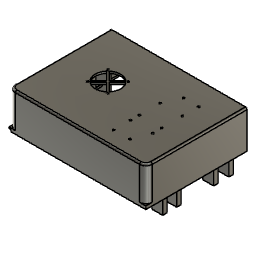
후방 상단 덮개 (Autodesk Fusion 360 design; units mm, degrees)
Autodesk Fusion 360 part; units mm, degrees
note: some values were not read from the file. Set by a fixed rule: which sketch regions a step uses.
sketch "스케치1" plane through (0, 0, 0) normal (0, 0, 1) x (1, 0, 0)
  line L0 (107.5, 79.5) -> (-107.5, 79.5)
  line L1 (-107.5, 79.5) -> (-107.5, -79.5)
  line L2 (-107.5, -79.5) -> (107.5, -79.5)
  line L3 (107.5, -79.5) -> (107.5, 79.5)
  line L4 (107.5, 79.5) -> (-107.5, -79.5) construction
  line L5 (-107.5, 79.5) -> (107.5, -79.5) construction
  line L6 (-107.5, 79.5) -> (-87.5, 79.5)
  line L7 (-87.5, 79.5) -> (-87.5, -79.5)
  line L8 (-87.5, -79.5) -> (-107.5, -79.5)
  line L9 (-107.5, -79.5) -> (-107.5, 79.5)
  line L10 (107.5, 79.5) -> (87.5, 79.5)
  line L11 (87.5, 79.5) -> (87.5, -79.5)
  line L12 (87.5, -79.5) -> (107.5, -79.5)
  line L13 (107.5, -79.5) -> (107.5, 79.5)
  line L14 (-107.5, 79.5) -> (-107.5, 69.5)
  line L15 (0, 0) -> (0, 10)
  line L16 (-107.5, 69.5) -> (-87.5, 69.5)
  line L17 (-87.5, 69.5) -> (-87.5, 21.5)
  line L18 (-87.5, 21.5) -> (-107.5, 21.5)
  line L19 (-107.5, 21.5) -> (-107.5, 69.5)
  line L20 (-97.5, 45.5) -> (-97.5, 57.5)
  line L21 (-107.5, 61) -> (-87.5, 61)
  line L22 (-87.5, 61) -> (-87.5, 54)
  line L23 (-87.5, 54) -> (-107.5, 54)
  line L24 (-107.5, 54) -> (-107.5, 61)
  line L25 (-107.5, 61) -> (-87.5, 54) construction
  line L26 (-87.5, 61) -> (-107.5, 54) construction
  line L27 (-97.5, 45.5) -> (-97.5, 33.5)
  line L28 (-87.5, 37) -> (-107.5, 37)
  line L29 (-107.5, 37) -> (-107.5, 30)
  line L30 (-107.5, 30) -> (-87.5, 30)
  line L31 (-87.5, 30) -> (-87.5, 37)
  line L32 (-87.5, 37) -> (-107.5, 30) construction
  line L33 (-107.5, 37) -> (-87.5, 30) construction
  circle A0 centre (-97.5, 57.5) radius 1.6
  circle A1 centre (-97.5, 33.5) radius 1.6
  line L34 (-107.5, -79.5) -> (-107.5, -59.5)
  line L35 (-107.5, -59.5) -> (-87.5, -59.5)
  line L36 (-87.5, -59.5) -> (-87.5, -11.5)
  line L37 (-87.5, -11.5) -> (-107.5, -11.5)
  line L38 (-107.5, -11.5) -> (-107.5, -59.5)
  line L39 (-97.5, -35.5) -> (-97.5, -24.5)
  line L40 (-97.5, -35.5) -> (-97.5, -46.5)
  line L41 (-107.5, -21) -> (-87.5, -21)
  line L42 (-87.5, -21) -> (-87.5, -28)
  line L43 (-87.5, -28) -> (-107.5, -28)
  line L44 (-107.5, -28) -> (-107.5, -21)
  line L45 (-107.5, -21) -> (-87.5, -28) construction
  line L46 (-87.5, -21) -> (-107.5, -28) construction
  line L47 (-87.5, -43) -> (-107.5, -43)
  line L48 (-107.5, -43) -> (-107.5, -50)
  line L49 (-107.5, -50) -> (-87.5, -50)
  line L50 (-87.5, -50) -> (-87.5, -43)
  line L51 (-87.5, -43) -> (-107.5, -50) construction
  line L52 (-107.5, -43) -> (-87.5, -50) construction
  circle A2 centre (-97.5, -24.5) radius 1.6
  circle A3 centre (-97.5, -46.5) radius 1.6
  line L53 (107.5, 79.5) -> (104.5, 79.5)
  line L54 (104.5, 79.5) -> (104.5, 76.5)
  line L55 (104.5, 76.5) -> (107.5, 76.5)
  line L56 (107.5, 76.5) -> (107.5, 79.5)
  line L57 (-107.5, -79.5) -> (-104.5, -79.5)
  line L58 (-104.5, -79.5) -> (-104.5, -76.5)
  line L59 (-104.5, -76.5) -> (-107.5, -76.5)
  line L60 (-107.5, -76.5) -> (-107.5, -79.5)
  line L61 (-104.5, -76.5) -> (104.5, -76.5)
  line L62 (104.5, -76.5) -> (104.5, 76.5)
  line L63 (104.5, 76.5) -> (-104.5, 76.5)
  line L64 (-104.5, 76.5) -> (-104.5, -76.5)
  line L65 (107.5, 61) -> (87.5, 61)
  line L66 (87.5, 61) -> (87.5, 54)
  line L67 (87.5, 54) -> (107.5, 54)
  line L68 (107.5, 54) -> (107.5, 61)
  circle A4 centre (97.5, 57.5) radius 1.6
  line L69 (107.5, 30) -> (87.5, 30)
  line L70 (87.5, 30) -> (87.5, 37)
  line L71 (107.5, 37) -> (107.5, 30)
  line L72 (87.5, 37) -> (107.5, 37)
  circle A5 centre (97.5, 33.5) radius 1.6
  line L73 (107.5, -50) -> (87.5, -50)
  line L74 (87.5, -50) -> (87.5, -43)
  line L75 (107.5, -43) -> (107.5, -50)
  line L76 (87.5, -43) -> (107.5, -43)
  circle A6 centre (97.5, -46.5) radius 1.6
  line L77 (107.5, -21) -> (87.5, -21)
  line L78 (87.5, -21) -> (87.5, -28)
  line L79 (107.5, -28) -> (107.5, -21)
  line L80 (87.5, -28) -> (107.5, -28)
  circle A7 centre (97.5, -24.5) radius 1.6
  line L81 (-104.5, 76.5) -> (-104.5, 79.5)
  point P0 (-97.5, 57.5)
  point P1 (-97.5, 33.5)
  point P2 (-97.5, -24.5)
  point P3 (-97.5, -46.5)
  dimension "d1" = 215
  dimension "d2" = 159
  dimension "d3" = 20
  dimension "d4" = 20
  dimension "d5" = 10
  dimension "d6" = 48
  dimension "d7" = 12
  dimension "d8" = 7
  dimension "d9" = 12
  dimension "d10" = 7
  dimension "d11" = 3.2
  dimension "d12" = 3.2
  dimension "d13" = 20
  dimension "d14" = 48
  dimension "d15" = 11
  dimension "d16" = 11
  dimension "d17" = 7
  dimension "d18" = 7
  dimension "d19" = 3.2
  dimension "d20" = 3.2
  dimension "d21" = 3
  dimension "d22" = 3
  dimension "d23" = 3
  dimension "d24" = 3
  constraint horizontal L0
  constraint perpendicular L0 L1
  constraint parallel L0 L2
  constraint parallel L1 L3
  constraint coincident L4 L15.start
  constraint coincident L5 L15.start
  constraint coincident L15.start origin
  constraint horizontal L6
  constraint vertical L7
  constraint horizontal L8
  constraint vertical L9
  constraint coincident L2 L7.end
  constraint horizontal L10
  constraint vertical L11
  constraint horizontal L12
  constraint vertical L13
  constraint perpendicular L6 L14
  constraint parallel L7 L15
  constraint horizontal L16
  constraint vertical L17
  constraint horizontal L18
  constraint vertical L19
  constraint perpendicular L18 L20
  constraint horizontal L21
  constraint perpendicular L21 L22
  constraint parallel L21 L23
  constraint parallel L22 L24
  constraint coincident L25 P0
  constraint coincident L26 P0
  constraint coincident P0 L20.end
  constraint parallel L20 L27
  constraint horizontal L28
  constraint perpendicular L28 L29
  constraint parallel L28 L30
  constraint parallel L29 L31
  constraint coincident L32 P1
  constraint coincident L33 P1
  constraint coincident P1 L27.end
  constraint perpendicular L2 L34
  constraint horizontal L35
  constraint vertical L36
  constraint horizontal L37
  constraint vertical L38
  constraint perpendicular L35 L39
  constraint perpendicular L37 L40
  constraint horizontal L41
  constraint perpendicular L41 L42
  constraint parallel L41 L43
  constraint parallel L42 L44
  constraint coincident L45 P2
  constraint coincident L46 P2
  constraint coincident P2 L39.end
  constraint horizontal L47
  constraint perpendicular L47 L48
  constraint parallel L47 L49
  constraint parallel L48 L50
  constraint coincident L51 P3
  constraint coincident L52 P3
  constraint coincident P3 L40.end
  constraint horizontal L53
  constraint vertical L54
  constraint horizontal L55
  constraint vertical L56
  constraint horizontal L57
  constraint vertical L58
  constraint horizontal L59
  constraint vertical L60
  constraint horizontal L61
  constraint vertical L62
  constraint horizontal L63
  constraint vertical L64
  constraint symmetric L15 L21.start L65.start
  constraint symmetric L15 L21.end L65.end
  constraint symmetric L15 L22.end L66.end
  constraint symmetric L15 L23.end L67.end
  constraint symmetric L15 L28.start L70.end
  constraint symmetric L15 L28.end L71.start
  constraint symmetric L15 L29.end L69.start
  constraint symmetric L15 L30.end L69.end
  constraint symmetric L15 A0 A4
  constraint symmetric L15 A1 A5
  constraint symmetric L15 L41.start L77.start
  constraint symmetric L15 L41.end L77.end
  constraint symmetric L15 L42.end L78.end
  constraint symmetric L15 L43.end L79.start
  constraint symmetric L15 L47.start L74.end
  constraint symmetric L15 L47.end L75.start
  constraint symmetric L15 L48.end L73.start
  constraint symmetric L15 L49.end L73.end
  constraint symmetric L15 A2 A7
  constraint symmetric L15 A3 A6
  constraint coincident L6 L81.end
  measures "d1" distance of L1.end L2.end
  measures "d2" distance of L0.end L1.end
  measures "d3" distance of L0.end L6.end
  measures "d4" distance of L0.start L10.end
  measures "d5" distance of L0.end L14.end
  measures "d6" distance of L14.end L18.end
  measures "d7" distance of L20.start P0
  measures "d8" distance of L21.end L22.end
  measures "d9" distance of L20.start P1
  measures "d10" distance of L28.end L29.end
  measures "d11" diameter of A0
  measures "d12" diameter of A1
  measures "d13" distance of L1.end L34.end
  measures "d14" distance of L34.end L37.end
  measures "d15" distance of L39.start P2
  measures "d16" distance of L39.start P3
  measures "d17" distance of L41.end L42.end
  measures "d18" distance of L47.end L48.end
  measures "d19" diameter of A2
  measures "d20" diameter of A3
  measures "d21" distance of L0.start L53.end
  measures "d22" distance of L0.start L55.end
  measures "d23" distance of L1.end L57.end
  measures "d24" distance of L1.end L59.end
extrude "돌출1" add sketch "스케치1" along normal blind 59 contours L0 L3 L10 L13 L53 L54 L55 L56 | L3 L13 L55 L62 L65 | L3 L13 L62 L65 L67 L68 | L3 L13 L62 L67 L72 | L0 L1 L6 L9 L14 L16 L64 L81 | L3 L13 L62 L69 L71 L72 | L3 L13 L62 L69 L77 | L1 L9 L16 L19 L21 L64 | L3 L13 L62 L77 L79 L80 | L1 L9 L19 L21 L23 L24 L64 | L3 L13 L62 L76 L80 | L1 L9 L19 L23 L28 L64 | L3 L13 L62 L73 L75 L76 | L1 L9 L19 L28 L29 L30 L64 | L2 L3 L11 L12 L13 L61 L62 L73 | L1 L9 L18 L19 L30 L64 | L1 L9 L18 L37 L64 | L2 L7 L11 L61 | L1 L9 L37 L38 L41 L64 | L2 L7 L8 L58 L61 | L1 L9 L38 L41 L43 L44 L64 | L1 L2 L8 L9 L34 L57 L58 L59 L60 | L1 L9 L38 L43 L47 L64 | L1 L9 L34 L35 L59 L64 | L1 L9 L38 L47 L48 L49 L64 | L1 L9 L35 L38 L49 L64
sketch "스케치2" plane through (0, 0, 0) normal (0, 0, -1) x (1, 0, 0)
  line L0 (-104.5, -76.5) -> (-104.5, 76.5)
  line L1 (-104.5, 76.5) -> (104.5, 76.5)
  line L2 (104.5, 76.5) -> (104.5, -79.5)
  line L3 (104.5, -79.5) -> (107.5, -79.5)
  line L4 (107.5, -79.5) -> (107.5, 79.5)
  line L5 (107.5, 79.5) -> (-107.5, 79.5)
  line L6 (-107.5, 79.5) -> (-107.5, -79.5)
  line L7 (-107.5, -79.5) -> (-104.5, -79.5)
  line L8 (-104.5, -79.5) -> (-104.5, -76.5)
  line L9 (-104.5, 76.5) -> (-94.5, 76.5)
  line L10 (-94.5, 76.5) -> (-94.5, -79.5)
  line L11 (-94.5, -79.5) -> (-104.5, -79.5)
  line L12 (-104.5, -79.5) -> (-104.5, 76.5)
  line L13 (104.5, 76.5) -> (94.5, 76.5)
  line L14 (94.5, 76.5) -> (94.5, -79.5)
  line L15 (94.5, -79.5) -> (104.5, -79.5)
  line L16 (104.5, -79.5) -> (104.5, 76.5)
  dimension "d27" = 10
  dimension "d28" = 10
  constraint horizontal L9
  constraint vertical L10
  constraint horizontal L11
  constraint vertical L12
  constraint coincident L0.end L1.start
  constraint horizontal L13
  constraint vertical L14
  constraint horizontal L15
  constraint vertical L16
  constraint coincident L1.end L2.start
  measures "d27" distance of L0.end L9.end
  measures "d28" distance of L1.end L13.end
extrude "돌출2" add sketch "스케치2" against normal blind 3 contours L0 L1 L8 L9 L10 L11 L12 | L1 L2 L13 L14 L15 L16
extrude "돌출3" add sketch "스케치1" against normal blind 24 contours L11 L62 L65 L66 L67 | L11 L62 L69 L70 L72 | L7 L17 L21 L22 L23 L64 | L11 L62 L77 L78 L80 | L7 L17 L28 L30 L31 L64 | L11 L62 L73 L74 L76 | L7 L36 L41 L42 L43 L64 | L7 L36 L47 L49 L50 L64
extrude "돌출4" add sketch "스케치1" against normal blind 21.8 contours A0 | A1 | A2 | A3 | A4 | A5 | A6 | A7
sketch "스케치3" plane through (104.5, 0, 0) normal (-1, 0, 0) x (0, -1, 0)
  line L0 (-79.5, 3) -> (76.5, 3)
  line L1 (76.5, 3) -> (76.5, 59)
  line L2 (76.5, 59) -> (-79.5, 59)
  line L3 (-79.5, 59) -> (-79.5, 3)
  line L4 (76.5, 59) -> (-79.5, 59)
  line L5 (-79.5, 59) -> (-79.5, 56)
  line L6 (-79.5, 56) -> (76.5, 56)
  line L7 (76.5, 56) -> (76.5, 59)
  dimension "d35" = 3
  constraint horizontal L4
  constraint vertical L5
  constraint horizontal L6
  constraint vertical L7
  constraint coincident L1.end L2.start
  measures "d35" distance of L1.end L6.end
extrude "돌출5" add sketch "스케치3" along normal blind 212 contours L1 L2 L3 L4 L5 L6 L7
extrude "돌출6" add 8 faces at (89.8333, 58.6667, 0) (89.8333, 34.6667, 0) (92.1667, -23.3333, 0) (92.1667, -47.6667, 0) (-89.8333, 58.6667, 0) (-89.8333, 32.3333, 0) (-92.1667, -45.3333, 0) (-92.1667, -25.6667, 0) along direction (0, 0, 1) blind 3
sketch "스케치6" plane through (0, 0, 3) normal (0, 0, 1) x (-1, 0, 0)
  line L0 (94.5, -79.5) -> (104.5, -79.5)
  line L1 (104.5, -79.5) -> (104.5, -76.5)
  line L2 (104.5, -76.5) -> (104.5, 76.5)
  line L3 (104.5, 76.5) -> (94.5, 76.5)
  line L4 (94.5, 76.5) -> (94.5, 50)
  line L5 (94.5, 50) -> (87.5, 50)
  line L6 (87.5, 50) -> (87.5, 43)
  line L7 (87.5, 43) -> (94.5, 43)
  line L8 (94.5, 43) -> (94.5, 28)
  line L9 (94.5, 28) -> (87.5, 28)
  line L10 (87.5, 28) -> (87.5, 21)
  line L11 (87.5, 21) -> (94.5, 21)
  line L12 (94.5, 21) -> (94.5, -30)
  line L13 (94.5, -30) -> (87.5, -30)
  line L14 (87.5, -30) -> (87.5, -37)
  line L15 (87.5, -37) -> (94.5, -37)
  line L16 (94.5, -37) -> (94.5, -54)
  line L17 (94.5, -54) -> (87.5, -54)
  line L18 (87.5, -54) -> (87.5, -61)
  line L19 (87.5, -61) -> (94.5, -61)
  line L20 (94.5, -61) -> (94.5, -79.5)
  line L21 (87.5, 50) -> (104.5, 50)
  line L22 (104.5, 50) -> (104.5, 43)
  line L23 (104.5, 43) -> (87.5, 43)
  line L24 (87.5, 43) -> (87.5, 50)
  line L25 (87.5, 28) -> (104.5, 28)
  line L26 (104.5, 28) -> (104.5, 21)
  line L27 (104.5, 21) -> (87.5, 21)
  line L28 (87.5, 21) -> (87.5, 28)
  line L29 (87.5, -30) -> (104.5, -30)
  line L30 (104.5, -30) -> (104.5, -37)
  line L31 (104.5, -37) -> (87.5, -37)
  line L32 (87.5, -37) -> (87.5, -30)
  line L33 (87.5, -54) -> (104.5, -54)
  line L34 (104.5, -54) -> (104.5, -61)
  line L35 (104.5, -61) -> (87.5, -61)
  line L36 (87.5, -61) -> (87.5, -54)
  dimension "d57" = 7
  dimension "d58" = 7
  dimension "d59" = 7
  dimension "d60" = 7
  constraint horizontal L21
  constraint vertical L22
  constraint horizontal L23
  constraint vertical L24
  constraint coincident L5.end L6.start
  constraint horizontal L25
  constraint vertical L26
  constraint horizontal L27
  constraint vertical L28
  constraint coincident L9.end L10.start
  constraint horizontal L29
  constraint vertical L30
  constraint horizontal L31
  constraint vertical L32
  constraint coincident L13.end L14.start
  constraint horizontal L33
  constraint vertical L34
  constraint horizontal L35
  constraint vertical L36
  constraint coincident L17.end L18.start
  measures "d57" distance of L5.end L6.end
  measures "d58" distance of L9.end L10.end
  measures "d59" distance of L13.end L14.end
  measures "d60" distance of L17.end L18.end
extrude "돌출10" add sketch "스케치6" along normal blind 56 contours L2 L17 L18 L19 L33 L34 L35 L36 | L2 L13 L14 L15 L29 L30 L31 L32 | L2 L9 L10 L11 L25 L26 L27 L28 | L2 L5 L6 L7 L21 L22 L23 L24
sketch "스케치7" plane through (0, 0, 3) normal (0, 0, 1) x (-1, 0, 0)
  line L0 (-104.5, 76.5) -> (-104.5, -79.5)
  line L1 (-104.5, -79.5) -> (-94.5, -79.5)
  line L2 (-94.5, -79.5) -> (-94.5, -61)
  line L3 (-94.5, -61) -> (-87.5, -61)
  line L4 (-87.5, -61) -> (-87.5, -54)
  line L5 (-87.5, -54) -> (-94.5, -54)
  line L6 (-94.5, -54) -> (-94.5, -37)
  line L7 (-94.5, -37) -> (-87.5, -37)
  line L8 (-87.5, -37) -> (-87.5, -30)
  line L9 (-87.5, -30) -> (-94.5, -30)
  line L10 (-94.5, -30) -> (-94.5, 21)
  line L11 (-94.5, 21) -> (-87.5, 21)
  line L12 (-87.5, 21) -> (-87.5, 28)
  line L13 (-87.5, 28) -> (-94.5, 28)
  line L14 (-94.5, 28) -> (-94.5, 43)
  line L15 (-94.5, 43) -> (-87.5, 43)
  line L16 (-87.5, 43) -> (-87.5, 50)
  line L17 (-87.5, 50) -> (-94.5, 50)
  line L18 (-94.5, 50) -> (-94.5, 76.5)
  line L19 (-94.5, 76.5) -> (-104.5, 76.5)
  line L20 (-87.5, 50) -> (-104.5, 50)
  line L21 (-104.5, 50) -> (-104.5, 43)
  line L22 (-104.5, 43) -> (-87.5, 43)
  line L23 (-87.5, 43) -> (-87.5, 50)
  line L24 (-87.5, 28) -> (-104.5, 28)
  line L25 (-104.5, 28) -> (-104.5, 21)
  line L26 (-104.5, 21) -> (-87.5, 21)
  line L27 (-87.5, 21) -> (-87.5, 28)
  line L28 (-87.5, -30) -> (-104.5, -30)
  line L29 (-104.5, -30) -> (-104.5, -37)
  line L30 (-104.5, -37) -> (-87.5, -37)
  line L31 (-87.5, -37) -> (-87.5, -30)
  line L32 (-87.5, -54) -> (-104.5, -54)
  line L33 (-104.5, -54) -> (-104.5, -61)
  line L34 (-104.5, -61) -> (-87.5, -61)
  line L35 (-87.5, -61) -> (-87.5, -54)
  dimension "d63" = 7
  dimension "d64" = 7
  dimension "d65" = 17
  dimension "d66" = 7
  dimension "d67" = 7
  constraint horizontal L20
  constraint vertical L21
  constraint horizontal L22
  constraint vertical L23
  constraint coincident L16.end L17.start
  constraint horizontal L24
  constraint vertical L25
  constraint horizontal L26
  constraint vertical L27
  constraint coincident L12.end L13.start
  constraint horizontal L28
  constraint vertical L29
  constraint horizontal L30
  constraint vertical L31
  constraint coincident L8.end L9.start
  constraint horizontal L32
  constraint vertical L33
  constraint horizontal L34
  constraint vertical L35
  constraint coincident L4.end L5.start
  measures "d63" distance of L16.end L15.end
  measures "d64" distance of L12.end L11.end
  measures "d65" distance of L8.end L28.end
  measures "d66" distance of L8.end L7.end
  measures "d67" distance of L4.end L3.end
extrude "돌출11" add sketch "스케치7" along normal blind 56 contours L0 L15 L16 L17 L20 L21 L22 L23 | L0 L11 L12 L13 L24 L25 L26 L27 | L0 L7 L8 L9 L28 L29 L30 L31 | L0 L3 L4 L5 L32 L33 L34 L35
sketch "스케치4" plane through (0, 0, 0) normal (0, 0, -1) x (1, 0, 0)
  line L0 (104.5, 43) -> (94.5, 43)
  line L1 (94.5, 43) -> (94.5, 28)
  line L2 (94.5, 28) -> (104.5, 28)
  line L3 (104.5, 28) -> (104.5, 21)
  line L4 (104.5, 21) -> (94.5, 21)
  line L5 (94.5, 21) -> (94.5, -30)
  line L6 (94.5, -30) -> (104.5, -30)
  line L7 (104.5, -30) -> (104.5, -37)
  line L8 (104.5, -37) -> (94.5, -37)
  line L9 (94.5, -37) -> (94.5, -54)
  line L10 (94.5, -54) -> (104.5, -54)
  line L11 (104.5, -54) -> (104.5, -61)
  line L12 (104.5, -61) -> (94.5, -61)
  line L13 (94.5, -61) -> (94.5, -79.5)
  line L14 (94.5, -79.5) -> (107.5, -79.5)
  line L15 (107.5, -79.5) -> (107.5, 79.5)
  line L16 (107.5, 79.5) -> (-107.5, 79.5)
  line L17 (-107.5, 79.5) -> (-107.5, -79.5)
  line L18 (-107.5, -79.5) -> (-104.5, -79.5)
  line L19 (-104.5, -79.5) -> (-94.5, -79.5)
  line L20 (-94.5, -79.5) -> (-94.5, -61)
  line L21 (-94.5, -61) -> (-104.5, -61)
  line L22 (-104.5, -61) -> (-104.5, -54)
  line L23 (-104.5, -54) -> (-94.5, -54)
  line L24 (-94.5, -54) -> (-94.5, -37)
  line L25 (-94.5, -37) -> (-104.5, -37)
  line L26 (-104.5, -37) -> (-104.5, -30)
  line L27 (-104.5, -30) -> (-94.5, -30)
  line L28 (-94.5, -30) -> (-94.5, 21)
  line L29 (-94.5, 21) -> (-104.5, 21)
  line L30 (-104.5, 21) -> (-104.5, 28)
  line L31 (-104.5, 28) -> (-94.5, 28)
  line L32 (-94.5, 28) -> (-94.5, 43)
  line L33 (-94.5, 43) -> (-104.5, 43)
  line L34 (-104.5, 43) -> (-104.5, 50)
  line L35 (-104.5, 50) -> (-94.5, 50)
  line L36 (-94.5, 50) -> (-94.5, 76.5)
  line L37 (-94.5, 76.5) -> (94.5, 76.5)
  line L38 (94.5, 76.5) -> (94.5, 50)
  line L39 (94.5, 50) -> (104.5, 50)
  line L40 (104.5, 50) -> (104.5, 43)
  line L41 (-107.5, 79.5) -> (-97.5, 79.5)
  line L42 (-97.5, 79.5) -> (-97.5, 69.5)
  line L43 (-97.5, 69.5) -> (-107.5, 69.5)
  line L44 (-107.5, 69.5) -> (-107.5, 79.5)
  line L45 (107.5, 79.5) -> (97.5, 79.5)
  line L46 (97.5, 79.5) -> (97.5, 69.5)
  line L47 (97.5, 69.5) -> (107.5, 69.5)
  line L48 (107.5, 69.5) -> (107.5, 79.5)
  dimension "d44" = 10
  dimension "d45" = 10
  dimension "d46" = 10
  dimension "d47" = 10
  constraint horizontal L41
  constraint vertical L42
  constraint horizontal L43
  constraint vertical L44
  constraint coincident L16.end L17.start
  constraint horizontal L45
  constraint vertical L46
  constraint horizontal L47
  constraint vertical L48
  constraint coincident L15.end L16.start
  measures "d44" distance of L16.end L41.end
  measures "d45" distance of L16.end L43.end
  measures "d46" distance of L15.end L45.end
  measures "d47" distance of L15.end L47.end
extrude "돌출7" add sketch "스케치4" against normal blind 5 contours L15 L16 L45 L46 L47 L48 | L16 L17 L41 L42 L43 L44
extrude "돌출8" cut 2 faces at (-102.1667, -74.1667, 5) (99.8333, -74.1667, 5) along direction (0, 0, -1) blind 2
sketch "스케치8" plane through (0, 0, 3) normal (0, 0, 1) x (-1, 0, 0)
  line L0 (-104.5, 76.5) -> (-104.5, 50)
  line L1 (-104.5, 50) -> (-94.5, 50)
  line L2 (-94.5, 50) -> (-94.5, 76.5)
  line L3 (-94.5, 76.5) -> (-104.5, 76.5)
  line L4 (-104.5, 76.5) -> (-94.5, 76.5)
  line L5 (-94.5, 76.5) -> (-94.5, 71.5)
  line L6 (-94.5, 71.5) -> (-104.5, 71.5)
  line L7 (-104.5, 71.5) -> (-104.5, 76.5)
  dimension "d70" = 5
  constraint horizontal L4
  constraint vertical L5
  constraint horizontal L6
  constraint vertical L7
  constraint coincident L0.start L3.end
  measures "d70" distance of L0.start L6.end
sketch "스케치9" plane through (0, 0, 3) normal (0, 0, 1) x (-1, 0, 0)
  line L0 (104.5, 76.5) -> (94.5, 76.5)
  line L1 (94.5, 76.5) -> (94.5, 50)
  line L2 (94.5, 50) -> (104.5, 50)
  line L3 (104.5, 76.5) -> (94.5, 76.5)
  line L4 (94.5, 76.5) -> (94.5, 71.5)
  line L5 (94.5, 71.5) -> (104.5, 71.5)
  line L6 (104.5, 71.5) -> (104.5, 76.5)
  line L7 (104.5, 50) -> (104.5, 76.5)
  dimension "d71" = 5
  constraint horizontal L3
  constraint vertical L4
  constraint horizontal L5
  constraint vertical L6
  constraint coincident L0.start L3.start
  measures "d71" distance of L0.start L5.end
extrude "돌출12" add sketch "스케치9" sketch "스케치8" along normal blind 56 contours L0 L1 L3 L4 L5 L6 L7 of sketch 2 contours L0 L2 L3 L4 L5 L6 L7
sketch "스케치10" plane through (0, 0, 59) normal (0, 0, 1) x (-1, 0, 0)
  line L0 (107.5, -79.5) -> (107.5, 79.5)
  line L1 (107.5, 79.5) -> (-107.5, 79.5)
  line L2 (-107.5, 79.5) -> (-107.5, -79.5)
  line L3 (-107.5, -79.5) -> (107.5, -79.5)
  line L4 (107.5, -79.5) -> (37.5, -79.5)
  line L5 (37.5, -79.5) -> (37.5, -6)
  line L6 (37.5, -6) -> (107.5, -6)
  line L7 (107.5, -6) -> (107.5, -79.5)
  line L8 (21.5, 10) -> (53.5, 10)
  line L9 (53.5, 10) -> (53.5, -22)
  line L10 (53.5, -22) -> (21.5, -22)
  line L11 (21.5, -22) -> (21.5, 10)
  line L12 (21.5, 10) -> (53.5, -22) construction
  line L13 (53.5, 10) -> (21.5, -22) construction
  circle A0 centre (21.5, 10) radius 1.6
  circle A1 centre (21.5, -22) radius 1.6
  circle A2 centre (53.5, -22) radius 1.6
  circle A3 centre (53.5, 10) radius 1.6
  circle A4 centre (37.5, -6) radius 20
  line L14 (37.5, -6) -> (36.4393, -7.0607)
  line L15 (36.4393, -7.0607) -> (20.833, 8.5456)
  line L16 (37.5, -6) -> (38.5607, -4.9393)
  line L17 (38.5607, -4.9393) -> (22.9544, 10.667)
  line L18 (37.5, -6) -> (38.5607, -4.9393)
  line L19 (38.5607, -4.9393) -> (54.167, -20.5456)
  line L20 (37.5, -6) -> (36.4393, -7.0607)
  line L21 (36.4393, -7.0607) -> (52.0456, -22.667)
  line L22 (37.5, -6) -> (36.4393, -4.9393)
  line L23 (36.4393, -4.9393) -> (20.833, -20.5456)
  line L24 (37.5, -6) -> (38.5607, -7.0607)
  line L25 (38.5607, -7.0607) -> (22.9544, -22.667)
  line L26 (38.5607, -7.0607) -> (54.167, 8.5456)
  line L27 (37.5, -6) -> (38.5607, -7.0607)
  line L28 (37.5, -6) -> (36.4393, -4.9393)
  line L29 (36.4393, -4.9393) -> (52.0456, 10.667)
  point P0 (37.5, -6)
  dimension "d74" = 70
  dimension "d75" = 73.5
  dimension "d76" = 32
  dimension "d77" = 32
  dimension "d78" = 3.2
  dimension "d79" = 3.2
  dimension "d80" = 3.2
  dimension "d81" = 3.2
  dimension "d82" = 40
  dimension "d96" = 1.5
  dimension "d97" = 1.5
  dimension "d98" = 1.5
  dimension "d99" = 1.5
  constraint horizontal L4
  constraint vertical L5
  constraint horizontal L6
  constraint vertical L7
  constraint coincident L0.start L3.end
  constraint horizontal L8
  constraint perpendicular L8 L9
  constraint parallel L8 L10
  constraint parallel L9 L11
  constraint coincident L12 P0
  constraint coincident L13 P0
  constraint coincident P0 L5.end
  constraint coincident L8.start L11.end
  constraint coincident L10.end L11.start
  constraint coincident L9.end L10.start
  constraint coincident L8.end L9.start
  constraint parallel L13 L14
  constraint coincident A0 L15.end
  constraint perpendicular L14 L15
  constraint perpendicular L12 L16
  constraint coincident A0 L17.end
  constraint perpendicular L13 L17
  constraint symmetric P0 L14 L5.end
  constraint symmetric L15.start L14 L20.end
  constraint symmetric L14 L15.end L21.end
  constraint symmetric L14 P0 L5.end
  constraint symmetric L14 L16.end L17.start
  constraint symmetric L14 L17.end L19.end
  constraint perpendicular L18 L22
  constraint coincident A1 L23.end
  constraint perpendicular L22 L23
  constraint perpendicular L18 L24
  constraint coincident A1 L25.end
  constraint perpendicular L24 L25
  constraint symmetric P0 L22 L5.end
  constraint symmetric L23.start L22 L28.end
  constraint symmetric L22 L23.end L29.end
  constraint symmetric L22 L24.end L25.start
  constraint symmetric L22 L25.end L26.end
  measures "d74" distance of L0.start L4.end
  measures "d75" distance of L0.start L6.end
  measures "d76" distance of L9.end L10.end
  measures "d77" distance of L8.end L9.end
  measures "d78" diameter of A0
  measures "d79" diameter of A1
  measures "d80" diameter of A2
  measures "d81" diameter of A3
  measures "d82" diameter of A4
  measures "d96" distance of P0 L14.end
  measures "d97" distance of P0 L16.end
  measures "d98" distance of P0 L22.end
  measures "d99" distance of P0 L24.end
extrude "돌출13" cut sketch "스케치10" against normal blind 3 contours L6 L9 A4 | L6 L9 A4 | L5 L10 A4 | L5 L10 A4 | L6 L9 A4 L19 | L6 L9 A4 L26 | L5 L10 A4 L25 | L5 L10 A4 L21 | L8 L9 A3 | L8 L9 A3 | L8 A4 L17 L29 | L9 L10 A2 | L9 L10 A2 | L10 L11 A1 | L10 L11 A1 | L11 A4 L15 L23 | L8 A4 | L11 A4 | L8 L11 A0 | L8 L11 A0
fillet "필렛4" radius 2.5 3 edges at (-107.5, 0, 59) (0, -79.5, 59) (107.5, 0, 59)
fillet "필렛5" radius 10 4 edges at (-107.5, -79.5, 28.25) (-106.7678, -78.7678, 58.2678) (107.5, -79.5, 28.25) (106.7678, -78.7678, 58.2678)
sketch "스케치11" plane through (0, 0, 0) normal (0, 0, -1) x (1, 0, 0)
  arc A0 (107.5, 69.5) -> (97.5, 79.5) centre (97.5, 69.5) ccw
  line L0 (97.5, 79.5) -> (-97.5, 79.5)
  arc A1 (-97.5, 79.5) -> (-107.5, 69.5) centre (-97.5, 69.5) ccw
  line L1 (-107.5, 69.5) -> (-107.5, -79.5)
  line L2 (-107.5, -79.5) -> (-104.5, -79.5)
  line L3 (-104.5, -79.5) -> (-94.5, -79.5)
  line L4 (-94.5, -79.5) -> (-94.5, -61)
  line L5 (-94.5, -61) -> (-104.5, -61)
  line L6 (-104.5, -61) -> (-104.5, -54)
  line L7 (-104.5, -54) -> (-94.5, -54)
  line L8 (-94.5, -54) -> (-94.5, -37)
  line L9 (-94.5, -37) -> (-104.5, -37)
  line L10 (-104.5, -37) -> (-104.5, -30)
  line L11 (-104.5, -30) -> (-94.5, -30)
  line L12 (-94.5, -30) -> (-94.5, 21)
  line L13 (-94.5, 21) -> (-104.5, 21)
  line L14 (-104.5, 21) -> (-104.5, 28)
  line L15 (-104.5, 28) -> (-94.5, 28)
  line L16 (-94.5, 28) -> (-94.5, 43)
  line L17 (-94.5, 43) -> (-104.5, 43)
  line L18 (-104.5, 43) -> (-104.5, 50)
  line L19 (-104.5, 50) -> (-94.5, 50)
  line L20 (-94.5, 50) -> (-94.5, 76.5)
  line L21 (-94.5, 76.5) -> (94.5, 76.5)
  line L22 (94.5, 76.5) -> (94.5, 50)
  line L23 (94.5, 50) -> (104.5, 50)
  line L24 (104.5, 50) -> (104.5, 43)
  line L25 (104.5, 43) -> (94.5, 43)
  line L26 (94.5, 43) -> (94.5, 28)
  line L27 (94.5, 28) -> (104.5, 28)
  line L28 (104.5, 28) -> (104.5, 21)
  line L29 (104.5, 21) -> (94.5, 21)
  line L30 (94.5, 21) -> (94.5, -30)
  line L31 (94.5, -30) -> (104.5, -30)
  line L32 (104.5, -30) -> (104.5, -37)
  line L33 (104.5, -37) -> (94.5, -37)
  line L34 (94.5, -37) -> (94.5, -54)
  line L35 (94.5, -54) -> (104.5, -54)
  line L36 (104.5, -54) -> (104.5, -61)
  line L37 (104.5, -61) -> (94.5, -61)
  line L38 (94.5, -61) -> (94.5, -79.5)
  line L39 (94.5, -79.5) -> (107.5, -79.5)
  line L40 (107.5, -79.5) -> (107.5, 69.5)
  line L41 (-107.5, 79.5) -> (-94.5, 79.5)
  line L42 (-94.5, 79.5) -> (-94.5, 69.5)
  line L43 (-94.5, 69.5) -> (-107.5, 69.5)
  line L44 (-107.5, 69.5) -> (-107.5, 79.5)
  line L45 (107.5, 79.5) -> (94.5, 79.5)
  line L46 (94.5, 79.5) -> (94.5, 69.5)
  line L47 (94.5, 69.5) -> (107.5, 69.5)
  line L48 (107.5, 69.5) -> (107.5, 79.5)
  constraint horizontal L41
  constraint vertical L42
  constraint horizontal L43
  constraint vertical L44
  constraint coincident L20 L42.end
  constraint horizontal L45
  constraint vertical L46
  constraint horizontal L47
  constraint vertical L48
  constraint coincident L22 L46.end
extrude "돌출14" add sketch "스케치11" against normal blind 5 contours A0 L45 L48 | A1 L41 L44
sketch "스케치5" plane through (0, 0, 0) normal (0, 0, -1) x (1, 0, 0)
  line L0 (-107.5, 79.5) -> (-107.5, -79.5)
  line L1 (-107.5, -79.5) -> (-104.5, -79.5)
  line L2 (-104.5, -79.5) -> (-94.5, -79.5)
  line L3 (-94.5, -79.5) -> (-94.5, -61)
  line L4 (-94.5, -61) -> (-104.5, -61)
  line L5 (-104.5, -61) -> (-104.5, -54)
  line L6 (-104.5, -54) -> (-94.5, -54)
  line L7 (-94.5, -37) -> (-104.5, -37)
  line L8 (-104.5, -37) -> (-104.5, -30)
  line L9 (-104.5, -30) -> (-94.5, -30)
  line L10 (-94.5, 21) -> (-104.5, 21)
  line L11 (-104.5, 21) -> (-104.5, 28)
  line L12 (-104.5, 28) -> (-94.5, 28)
  line L13 (-94.5, 43) -> (-104.5, 43)
  line L14 (-104.5, 43) -> (-104.5, 50)
  line L15 (-104.5, 50) -> (-94.5, 50)
  line L16 (-94.5, 76.5) -> (94.5, 76.5)
  line L17 (94.5, 76.5) -> (94.5, 50)
  line L18 (94.5, 50) -> (104.5, 50)
  line L19 (104.5, 50) -> (104.5, 43)
  line L20 (104.5, 43) -> (94.5, 43)
  line L21 (94.5, 28) -> (104.5, 28)
  line L22 (104.5, 28) -> (104.5, 21)
  line L23 (104.5, 21) -> (94.5, 21)
  line L24 (94.5, -30) -> (104.5, -30)
  line L25 (104.5, -30) -> (104.5, -37)
  line L26 (104.5, -37) -> (94.5, -37)
  line L27 (94.5, -54) -> (104.5, -54)
  line L28 (104.5, -54) -> (104.5, -61)
  line L29 (104.5, -61) -> (94.5, -61)
  line L30 (94.5, -79.5) -> (107.5, -79.5)
  line L31 (107.5, -79.5) -> (107.5, 79.5)
  line L32 (107.5, 79.5) -> (-107.5, 79.5)
  line L33 (-107.5, 79.5) -> (-104.5, 79.5)
  line L34 (-104.5, 79.5) -> (-104.5, -20.5)
  line L35 (-104.5, -20.5) -> (-107.5, -20.5)
  line L36 (-107.5, -20.5) -> (-107.5, 79.5)
  line L37 (-94.5, -54) -> (-94.5, -37)
  line L38 (-94.5, -30) -> (-94.5, 21)
  line L39 (-94.5, 28) -> (-94.5, 43)
  line L40 (-94.5, 50) -> (-94.5, 76.5)
  line L41 (94.5, 43) -> (94.5, 28)
  line L42 (94.5, 21) -> (94.5, -30)
  line L43 (94.5, -37) -> (94.5, -54)
  line L44 (94.5, -61) -> (94.5, -79.5)
  dimension "d52" = 100
  constraint horizontal L33
  constraint vertical L34
  constraint horizontal L35
  constraint vertical L36
  constraint coincident L0.start L32.end
  measures "d52" distance of L0.start L35.end
extrude "돌출9" cut sketch "스케치5" against normal blind 3 contours L0 L11 L14 L32 L33 L34 L35 L36
fillet "필렛3" radius 1 1 edges at (-107.5, -29.5, 3)
sketch "스케치12" plane through (0, 0, 59) normal (0, 0, 1) x (-1, 0, 0)
  arc A0 (-97.5, 77) -> (-105, 69.5) centre (-97.5, 69.5) ccw
  line L0 (-105, 69.5) -> (-105, -79.5)
  line L1 (-105, -79.5) -> (105, -79.5)
  line L2 (105, -79.5) -> (105, 69.5)
  arc A1 (105, 69.5) -> (97.5, 77) centre (97.5, 69.5) ccw
  line L3 (97.5, 77) -> (-97.5, 77)
  circle A2 centre (21.5, 10) radius 1.6
  circle A3 centre (53.5, 10) radius 1.6
  circle A4 centre (21.5, -22) radius 1.6
  circle A5 centre (53.5, -22) radius 1.6
  line L4 (-82.5, 70) -> (-17.5, 70)
  line L5 (-17.5, 70) -> (-17.5, -70)
  line L6 (-17.5, -70) -> (-82.5, -70)
  line L7 (-82.5, -70) -> (-82.5, 70)
  line L8 (-82.5, 70) -> (-17.5, -70) construction
  line L9 (-17.5, 70) -> (-82.5, -70) construction
  line L10 (37.5, -3.8787) -> (24.4584, 9.163)
  arc A6 (50.5416, 9.163) -> (24.4584, 9.163) centre (37.5, -6) ccw
  line L11 (50.5416, 9.163) -> (37.5, -3.8787)
  line L12 (37.5, -8.1213) -> (50.5416, -21.163)
  arc A7 (24.4584, -21.163) -> (50.5416, -21.163) centre (37.5, -6) ccw
  line L13 (24.4584, -21.163) -> (37.5, -8.1213)
  arc A8 (52.663, -19.0416) -> (52.663, 7.0416) centre (37.5, -6) ccw
  line L14 (52.663, -19.0416) -> (39.6213, -6)
  line L15 (39.6213, -6) -> (52.663, 7.0416)
  arc A9 (22.337, 7.0416) -> (22.337, -19.0416) centre (37.5, -6) ccw
  line L16 (22.337, 7.0416) -> (35.3787, -6)
  line L17 (35.3787, -6) -> (22.337, -19.0416)
  line L18 (-82.5, -70) -> (-68, -70)
  line L19 (-68, -70) -> (-68, -43)
  line L20 (-68, -43) -> (-82.5, -43)
  line L21 (-82.5, -43) -> (-82.5, -70)
  circle A10 centre (-68, -43) radius 1.6
  line L22 (-68, -43) -> (-44.5, -43)
  circle A11 centre (-44.5, -43) radius 1.6
  line L23 (-68, -43) -> (-68, -17.5)
  circle A12 centre (-68, -17.5) radius 1.6
  line L24 (-68, -17.5) -> (-33, -17.5)
  circle A13 centre (-33, -17.5) radius 1.6
  line L25 (-68, -17.5) -> (-68, 15)
  circle A14 centre (-68, 15) radius 1.6
  line L26 (-68, 15) -> (-33, 15)
  circle A15 centre (-33, 15) radius 1.6
  line L27 (-68, 29) -> (-33, 29)
  circle A16 centre (-68, 29) radius 1.6
  circle A17 centre (-33, 29) radius 1.6
  line L28 (-68, 29) -> (-58, 29)
  line L29 (-58, 29) -> (-58, 55)
  line L30 (-58, 55) -> (-68, 55)
  line L31 (-68, 55) -> (-68, 29)
  circle A18 centre (-58, 55) radius 1.6
  line L32 (-33, 29) -> (-33, 55.5)
  circle A19 centre (-33, 55.5) radius 1.6
  point P0 (-50, 0)
  dimension "d91" = 65
  dimension "d92" = 140
  dimension "d104" = 3.2
  dimension "d105" = 3.2
  dimension "d106" = 23.5
  dimension "d107" = 25.5
  dimension "d108" = 3.2
  dimension "d109" = 3.2
  dimension "d110" = 3.2
  dimension "d111" = 3.2
  dimension "d112" = 3.2
  dimension "d113" = 3.2
  dimension "d114" = 3.2
  dimension "d115" = 26.5
  dimension "d116" = 3.2
  constraint horizontal L4
  constraint perpendicular L4 L5
  constraint parallel L4 L6
  constraint parallel L5 L7
  constraint coincident L8 P0
  constraint coincident L9 P0
  constraint horizontal L18
  constraint vertical L19
  constraint horizontal L20
  constraint vertical L21
  constraint coincident L19.end L20.start
  constraint perpendicular L19 L22
  constraint coincident L22.end A11.centre
  constraint parallel L19 L23
  constraint coincident L23.end A12.centre
  constraint horizontal L24
  constraint coincident L24.end A13.centre
  constraint perpendicular L24 L25
  constraint coincident L25.end A14.centre
  constraint perpendicular L25 L26
  constraint coincident L26.end A15.centre
  constraint parallel L26 L27
  constraint coincident L27.start A16.centre
  constraint coincident L27.end A17.centre
  constraint horizontal L28
  constraint vertical L29
  constraint horizontal L30
  constraint vertical L31
  constraint coincident L29.end L30.start
  constraint perpendicular L27 L32
  constraint coincident L32.end A19.centre
  measures "d91" distance of L5.end L6.end
  measures "d92" distance of L4.end L5.end
  measures "d104" diameter of A10
  measures "d105" diameter of A11
  measures "d106" distance of L19.end L22.end
  measures "d107" distance of L19.end L23.end
  measures "d108" diameter of A12
  measures "d109" diameter of A13
  measures "d110" diameter of A14
  measures "d111" diameter of A15
  measures "d112" diameter of A16
  measures "d113" diameter of A17
  measures "d114" diameter of A18
  measures "d115" distance of L27.end L32.end
  measures "d116" diameter of A19
extrude "돌출16" cut sketch "스케치12" against normal blind 3 contours L20 A10 L23 | L19 L20 A10 | L19 A10 L22 | A10 L22 L23 | A11 | L23 A12 L25 | L23 A12 L24 | A12 L24 L25 | A13 | L25 A14 L26 | L25 A14 L26 | A15 | L27 A16 L28 L31 | L27 A16 L28 L31 | L29 L30 A18 | L29 L30 A18 | L27 A17 L32 | L27 A17 L32 | A19
fillet "필렛6" [suppressed]
fillet "필렛7" [suppressed]
